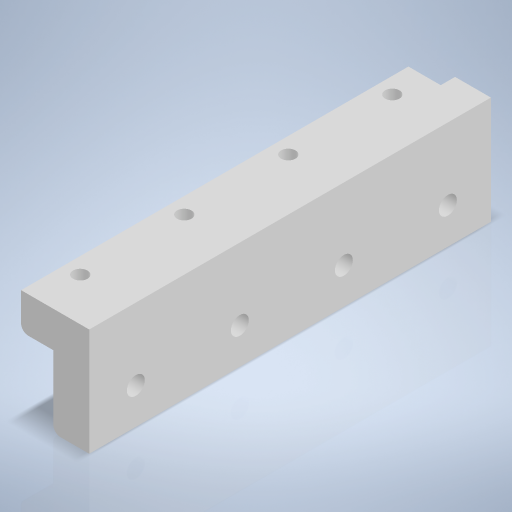
# Autodesk Inventor part: 1014_right
Saved by Autodesk Inventor 2024 (Build 280153000, 153)
## iProperties
Created: 2024-06-10
Part Number: 1014_right
Material: Generisch
Document SubType Name: Modeling
Designer: ffogue
Density: 1 g/cm^3
Appearance: Vorgabe
Author: ffogue
Autodesk Inventor part; units mm, degrees
ref_plane "YZ Plane" through (0, 0, 0) normal (1, 0, 0) x (0, 1, 0)
ref_plane "XZ Plane" through (0, 0, 0) normal (0, 1, 0) x (-1, 0, 0)
ref_plane "XY Plane" through (0, 0, 0) normal (0, 0, 1) x (1, 0, 0)
sketch "Skizze2" plane through (0, 0, 0) normal (0, 1, 0) x (-1, 0, 0)
  line L0 (0, 0) -> (19, 0)
  line L1 (19, 0) -> (19, -10)
  line L2 (19, -10) -> (10, -10)
  line L3 (10, -10) -> (10, -30)
  line L4 (10, -30) -> (0, -30)
  line L5 (0, -30) -> (0, 0)
  dimension "d6" = 10
  dimension "d7" = 20
  dimension "d8" = 10
  dimension "d9" = 9
  constraints: 12 end point, 5 perpendicular, 1 horizontal
  measures "d6" distance between parallel lines of L2 L0
  measures "d7" distance between parallel lines of L2 L4
  measures "d8" distance between parallel lines of L5 L3
  measures "d9" distance between parallel lines of L3 L1
extrude "Extrusion1" add sketch "Skizze2" along normal blind 112
sketch "Skizze3" plane through (-10, 0, -10) normal (0, 0, -1) x (-1, 0, 0)
  line L0 (0, 112) -> (9, 112) projected
  point P0 (-10, 0)
  point P1 (4.5, 99)
  point P2 (4.5, 70)
  point P3 (4.5, 41)
  point P4 (4.5, 12)
  point P5 (4.5, 112)
  point P6 (4.5, 112)
  dimension "d12" = 13
  dimension "d13" = 29
  dimension "d14" = 29
  dimension "d15" = 29
  constraints: 4 vertical alignment, 2 midpoint
  measures "d12" distance of point (4.5, 112) point (4.5, 99)
  measures "d13" distance of point (4.5, 70) point (4.5, 99)
  measures "d14" distance of point (4.5, 41) point (4.5, 70)
  measures "d15" distance of point (4.5, 12) point (4.5, 41)
hole "Bohrung1" at (-14.5, 99, -10) at (-14.5, 70, -10) at (-14.5, 41, -10) at (-14.5, 12, -10) direction (0, 0, 1) diameter 4 depth 10 countersink diameter 5 countersink angle 90
sketch "Skizze4" plane through (-10, 0, -30) normal (-1, 0, 0) x (0, 0, 1)
  line L0 (0, 112) -> (20, 112) projected
  line L1 (0, 0) -> (20, 0) projected
  point P0 (30, 0)
  point P1 (10, 100)
  point P2 (10, 71)
  point P3 (10, 42)
  point P4 (10, 13)
  point P5 (10, 0)
  dimension "d30" = 12
  dimension "d31" = 29
  dimension "d32" = 29
  dimension "d33" = 29
  constraints: 4 vertical alignment, 1 midpoint
  measures "d30" distance from line of L0 point (10, 100)
  measures "d31" distance of point (10, 71) point (10, 100)
  measures "d32" distance of point (10, 42) point (10, 71)
  measures "d33" distance of point (10, 13) point (10, 42)
hole "Bohrung2" at (-10, 100, -20) at (-10, 71, -20) at (-10, 42, -20) at (-10, 13, -20) direction (1, 0, 0) diameter 5 end through all
sketch "Skizze5" plane through (-10, 0, -10) normal (0, 0, -1) x (-1, 0, 0)
  line L0 (9, 112) -> (-0.0001, 112)
  line L1 (9, 112) -> (9, 108)
  line L2 (9, 0) -> (9, 112) projected
  line L3 (9, 108) -> (0, 108)
  line L4 (0, 0) -> (0, 112) projected
  line L5 (0, 112) -> (0, 108)
  point P0 (-10, 0)
  dimension "d40" = 4
  constraints: 8 end point, 2 point on line, 1 collinear, 1 horizontal, 1 perpendicular
  measures "d40" distance between parallel lines of L3 L0
extrude "Extrusion2" cut sketch "Skizze5" against normal up to surface (10 mm away)
fillet "Rundung1" radius 2 2 edges at (-10, 56, -30) (-19, 54, -10)
equation "\"d32\" = d31"
equation "\"d33\" = d32"
